Autodesk Fusion 360 part; units mm, degrees
(part 2 of 2)
sketch "Sketch10" plane through (0, -48, 0) normal (0, -1, 0) x (1, 0, 0)
  circle A0 centre (0, 0) radius 3
  line L0 (-36.294, 10) -> (-21.148, 10)
  arc A1 (-14.148, 3) -> (-21.148, 10) centre (-21.148, 3) ccw
  line L1 (-14.148, 3) -> (-14.148, -2.9712)
  arc A2 (-21.148, -9.9712) -> (-14.148, -2.9712) centre (-21.148, -2.9712) ccw
  line L2 (-21.148, -9.9712) -> (-36.294, -9.9712)
  arc A3 (-43.294, -2.9712) -> (-36.294, -9.9712) centre (-36.294, -2.9712) ccw
  line L3 (-43.294, -2.9712) -> (-43.294, 3)
  arc A4 (-36.294, 10) -> (-43.294, 3) centre (-36.294, 3) ccw
  circle A5 centre (0, 8.5) radius 3.05
  circle A6 centre (8.0981, 0) radius 3.05
  circle A7 centre (-8.0981, 0) radius 3.05
  circle A8 centre (0, -8.5) radius 3.05
  arc A9 (-41.8984, -20.1687) -> (-41.8984, 20.1687) centre (0, 0) ccw
  arc A10 (-37.3932, -13) -> (-41.8984, -20.1687) centre (-37.3932, -18) ccw
  line L4 (-37.3932, -13) -> (0, -13)
  arc A11 (0, -13) -> (0, 13) centre (0, 0) ccw
  line L5 (0, 13) -> (-37.3932, 13)
  arc A12 (-41.8984, 20.1687) -> (-37.3932, 13) centre (-37.3932, 18) ccw
  arc A13 (-50, 0.0217) -> (-50, -0.0217) centre (0, 0) ccw
  line L6 (-50, -0.0217) -> (-51.2179, -5.3832)
  line L7 (-51.2179, -5.3832) -> (-48.9119, -10.3743)
  arc A14 (-48.9119, -10.3743) -> (-48.9029, -10.4168) centre (0, 0) ccw
  line L8 (-48.9029, -10.4168) -> (-48.9794, -15.9144)
  line L9 (-48.9794, -15.9144) -> (-45.6861, -20.317)
  arc A15 (-45.6861, -20.317) -> (-45.6684, -20.3567) centre (0, 0) ccw
  line L10 (-45.6684, -20.3567) -> (-44.6003, -25.75)
  line L11 (-44.6003, -25.75) -> (-40.4636, -29.3717)
  arc A16 (-40.4636, -29.3717) -> (-40.4381, -29.4068) centre (0, 0) ccw
  line L12 (-40.4381, -29.4068) -> (-38.272, -34.4602)
  line L13 (-38.272, -34.4602) -> (-33.4727, -37.1427)
  arc A17 (-33.4727, -37.1427) -> (-33.4404, -37.1718) centre (0, 0) ccw
  line L14 (-33.4404, -37.1718) -> (-30.2709, -41.6644)
  line L15 (-30.2709, -41.6644) -> (-25.0188, -43.2904)
  arc A18 (-25.0188, -43.2904) -> (-24.9812, -43.3121) centre (0, 0) ccw
  line L16 (-24.9812, -43.3121) -> (-20.9469, -47.0476)
  line L17 (-20.9469, -47.0476) -> (-15.4715, -47.5461)
  arc A19 (-15.4715, -47.5461) -> (-15.4302, -47.5595) centre (0, 0) ccw
  line L18 (-15.4302, -47.5595) -> (-10.7075, -50.3746)
  line L19 (-10.7075, -50.3746) -> (-5.248, -49.7238)
  arc A20 (-5.248, -49.7238) -> (-5.2048, -49.7284) centre (0, 0) ccw
  line L20 (-5.2048, -49.7284) -> (0, -51.5)
  line L21 (0, -51.5) -> (5.2048, -49.7284)
  arc A21 (5.2048, -49.7284) -> (5.248, -49.7238) centre (0, 0) ccw
  line L22 (5.248, -49.7238) -> (10.7075, -50.3746)
  line L23 (10.7075, -50.3746) -> (15.4302, -47.5595)
  arc A22 (15.4302, -47.5595) -> (15.4715, -47.5461) centre (0, 0) ccw
  line L24 (15.4715, -47.5461) -> (20.9469, -47.0476)
  line L25 (20.9469, -47.0476) -> (24.9812, -43.3121)
  arc A23 (24.9812, -43.3121) -> (25.0188, -43.2904) centre (0, 0) ccw
  line L26 (25.0188, -43.2904) -> (30.2709, -41.6644)
  line L27 (30.2709, -41.6644) -> (33.4404, -37.1718)
  arc A24 (33.4404, -37.1718) -> (33.4727, -37.1427) centre (0, 0) ccw
  line L28 (33.4727, -37.1427) -> (38.272, -34.4602)
  line L29 (38.272, -34.4602) -> (40.4381, -29.4068)
  arc A25 (40.4381, -29.4068) -> (40.4636, -29.3717) centre (0, 0) ccw
  line L30 (40.4636, -29.3717) -> (44.6003, -25.75)
  line L31 (44.6003, -25.75) -> (45.6684, -20.3567)
  arc A26 (45.6684, -20.3567) -> (45.6861, -20.317) centre (0, 0) ccw
  line L32 (45.6861, -20.317) -> (48.9794, -15.9144)
  line L33 (48.9794, -15.9144) -> (48.9029, -10.4168)
  arc A27 (48.9029, -10.4168) -> (48.9119, -10.3743) centre (0, 0) ccw
  line L34 (48.9119, -10.3743) -> (51.2179, -5.3832)
  line L35 (51.2179, -5.3832) -> (50, -0.0217)
  arc A28 (50, -0.0217) -> (50, 0.0217) centre (0, 0) ccw
  line L36 (50, 0.0217) -> (51.2179, 5.3832)
  line L37 (51.2179, 5.3832) -> (48.9119, 10.3743)
  arc A29 (48.9119, 10.3743) -> (48.9029, 10.4168) centre (0, 0) ccw
  line L38 (48.9029, 10.4168) -> (48.9794, 15.9144)
  line L39 (48.9794, 15.9144) -> (45.6861, 20.317)
  arc A30 (45.6861, 20.317) -> (45.6684, 20.3567) centre (0, 0) ccw
  line L40 (45.6684, 20.3567) -> (44.6003, 25.75)
  line L41 (44.6003, 25.75) -> (40.4636, 29.3717)
  arc A31 (40.4636, 29.3717) -> (40.4381, 29.4068) centre (0, 0) ccw
  line L42 (40.4381, 29.4068) -> (38.272, 34.4602)
  line L43 (38.272, 34.4602) -> (33.4727, 37.1427)
  arc A32 (33.4727, 37.1427) -> (33.4404, 37.1718) centre (0, 0) ccw
  line L44 (33.4404, 37.1718) -> (30.2709, 41.6644)
  line L45 (30.2709, 41.6644) -> (25.0188, 43.2904)
  arc A33 (25.0188, 43.2904) -> (24.9812, 43.3121) centre (0, 0) ccw
  line L46 (24.9812, 43.3121) -> (20.9469, 47.0476)
  line L47 (20.9469, 47.0476) -> (15.4715, 47.5461)
  arc A34 (15.4715, 47.5461) -> (15.4302, 47.5595) centre (0, 0) ccw
  line L48 (15.4302, 47.5595) -> (10.7075, 50.3746)
  line L49 (10.7075, 50.3746) -> (5.248, 49.7238)
  arc A35 (5.248, 49.7238) -> (5.2048, 49.7284) centre (0, 0) ccw
  line L50 (5.2048, 49.7284) -> (0, 51.5)
  line L51 (0, 51.5) -> (-5.2048, 49.7284)
  arc A36 (-5.2048, 49.7284) -> (-5.248, 49.7238) centre (0, 0) ccw
  line L52 (-5.248, 49.7238) -> (-10.7075, 50.3746)
  line L53 (-10.7075, 50.3746) -> (-15.4302, 47.5595)
  arc A37 (-15.4302, 47.5595) -> (-15.4715, 47.5461) centre (0, 0) ccw
  line L54 (-15.4715, 47.5461) -> (-20.9469, 47.0476)
  line L55 (-20.9469, 47.0476) -> (-24.9812, 43.3121)
  arc A38 (-24.9812, 43.3121) -> (-25.0188, 43.2904) centre (0, 0) ccw
  line L56 (-25.0188, 43.2904) -> (-30.2709, 41.6644)
  line L57 (-30.2709, 41.6644) -> (-33.4404, 37.1718)
  arc A39 (-33.4404, 37.1718) -> (-33.4727, 37.1427) centre (0, 0) ccw
  line L58 (-33.4727, 37.1427) -> (-38.272, 34.4602)
  line L59 (-38.272, 34.4602) -> (-40.4381, 29.4068)
  arc A40 (-40.4381, 29.4068) -> (-40.4636, 29.3717) centre (0, 0) ccw
  line L60 (-40.4636, 29.3717) -> (-44.6003, 25.75)
  line L61 (-44.6003, 25.75) -> (-45.6684, 20.3567)
  arc A41 (-45.6684, 20.3567) -> (-45.6861, 20.317) centre (0, 0) ccw
  line L62 (-45.6861, 20.317) -> (-48.9794, 15.9144)
  line L63 (-48.9794, 15.9144) -> (-48.9029, 10.4168)
  arc A42 (-48.9029, 10.4168) -> (-48.9119, 10.3743) centre (0, 0) ccw
  line L64 (-48.9119, 10.3743) -> (-51.2179, 5.3832)
  line L65 (-51.2179, 5.3832) -> (-50, 0.0217)
  circle A43 centre (0, 0) radius 13
  constraint coincident A0.centre A9.centre
extrude "Extrude10" add sketch "Sketch10" against normal up to surface (16 mm away) contours A0 | A5 | A6 | A7 | A8 | A11 A43
sketch "Sketch11" plane through (0, -48, 0) normal (0, -1, 0) x (1, 0, 0)
  arc A0 (-1.7748, -1.9) -> (1.7748, -1.9) centre (0, 0) cw
  line L0 (1.7748, -1.9) -> (-1.7748, -1.9)
  arc A1 (1.8138, -2) -> (-1.8138, -2) centre (0, 0) ccw
  line L1 (1.8138, -2) -> (-1.8138, -2)
  dimension "d165" = -0.1
extrude "Extrude11" cut sketch "Sketch11" against normal up to surface (16 mm away) contours A0 L0 | A1 L1
